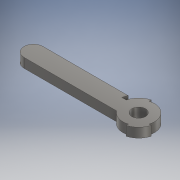
# Autodesk Inventor part: Handle Base Feature
Saved by Autodesk Inventor 2018 (Build 220112000, 112)
## iProperties
Created: 2017-09-07
Part Number: Handle Base Feature
Material: Steel, Mild
Document SubType Name: Modeling
Designer: kurtis
Density: 7.85 g/cm^3
Appearance: Semi-Polished
Author: kurtis
Autodesk Inventor part; units mm, degrees
ref_plane "YZ Plane" through (0, 0, 0) normal (1, 0, 0) x (0, 1, 0)
ref_plane "XZ Plane" through (0, 0, 0) normal (0, 1, 0) x (-1, 0, 0)
ref_plane "XY Plane" through (0, 0, 0) normal (0, 0, 1) x (1, 0, 0)
sketch "Sketch1" plane through (0, 0, 0) normal (0, 0, 1) x (1, 0, 0)
  circle A0 centre (0, 0) radius 6.5
  circle A1 centre (0, 0) radius 15
  arc A2 (-18.9737, 9) -> (-20.5122, 4.5) centre (0, 0) ccw
  arc A3 (-14.4222, -9) -> (-16.3936, 4.5) centre (0, 0) ccw
  line L0 (0, 17) -> (-4.5, 17) construction
  line L1 (17, 0) -> (17, -4.5) construction
  line L2 (16.3936, -4.5) -> (14.3091, -4.5)
  line L3 (0, -17) -> (4.5, -17) construction
  line L4 (4.5, -16.3936) -> (4.5, -14.3091)
  line L5 (-17, 0) -> (-17, 4.5) construction
  line L6 (-17, 4.5) -> (-14.3091, 4.5)
  line L7 (0, 0) -> (-100, 0) construction
  arc A4 (-100, 9) -> (-100, -9) centre (-100, 0) ccw
  line L8 (-100, -9) -> (-12, -9)
  line L9 (-100, 9) -> (-18.9737, 9)
  line L10 (-14.4222, 9) -> (-12, 9)
  line L11 (-17, 4.5) -> (-20.5122, 4.5)
  line L12 (-4.5, 16.3936) -> (-4.5, 14.3091)
  line L13 (-4.5, 16.3936) -> (-4.5, 17) construction
  line L14 (17, -4.5) -> (16.3936, -4.5) construction
  line L15 (4.5, -17) -> (4.5, -16.3936) construction
  dimension "d3" = 34
  dimension "d0" = 13
  dimension "d1" = 30
  dimension "d2" = 42
  dimension "d4" = 4.5
  dimension "d5" = 4.5
  dimension "d6" = 4.5
  dimension "d7" = 4.5
  dimension "d8" = 100
  dimension "d9" = 9
  constraints: 32 end point, 10 point on circle, 9 horizontal, 6 vertical, 5 coincident, 4 centre point, 3 perpendicular, 3 point on line, 3 tangent, 2 parallel, 1 collinear, 11 other
  measures "d0" diameter of A0
  measures "d1" diameter of A1
  measures "d2" diameter of A2
  measures "d4" distance of L0.start L0.end
  measures "d5" distance of L1.start L1.end
  measures "d6" distance of L3.start L3.end
  measures "d7" distance of L5.start L5.end
  measures "d8" distance of L7.start L7.end
  measures "d9" radius of A4
extrude "Extrusion1" add sketch "Sketch1" along normal blind 9 contours A1 | A1 L10 A3 L12 | L2 A3 L4 A1 | A1 L6 A3 L10 | A1 L8 A4 L9 A2 L11 L6
equation "\"d5\" = d4"
equation "\"d6\" = d4"
equation "\"d7\" = d4"
body "Solid1"
